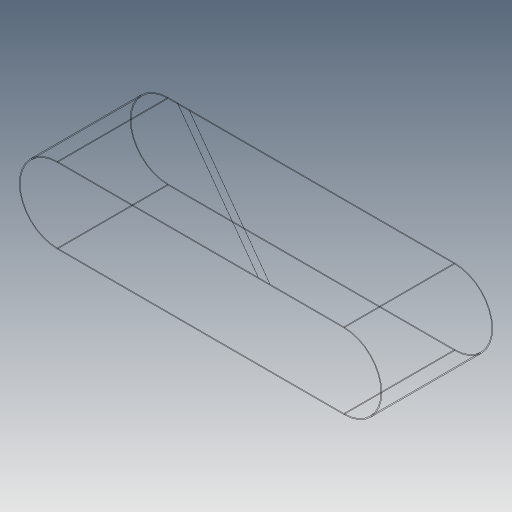
# Autodesk Inventor part: J005559
Saved by Autodesk Inventor 2023.3 (Build 273359000, 359)
## iProperties
RuleStatus: InUse
Created: 2015-04-28
Material: POLYESTER, BLACK
Vendor: HHMI: JRC - ID&F
Document SubType Name: Modeling
Designer: ARNOLDJ
Density: 1 g/cm^3
Appearance: Skid Plate
Description: RIBBON FLAT BELT
Project: COMMON
Part Number: J005559
AfterDocSave0: file://Part Number Cleaner
LAB/DEPT: COMMON
REQUESTING SCIENTIST: COMMON
SURFACE ROUGHNESS: N/A
DESIGN DEPARTMENT: HHMI: JRC - ID&F
SPECIAL FINISH: NONE
ALTERED ITEM PART NUMBER: SEE DRAWING
ALTERED ITEM VENDOR: SEE DRAWING
ALTERED ITEM DESCRIPTION: SEE DRAWING
Revision Number: B
Autodesk Inventor part; units mm, degrees
ref_plane "YZ Plane" through (0, 0, 0) normal (1, 0, 0) x (0, 1, 0)
ref_plane "XZ Plane" through (0, 0, 0) normal (0, 1, 0) x (-1, 0, 0)
ref_plane "XY Plane" through (0, 0, 0) normal (0, 0, 1) x (1, 0, 0)
sketch "Sketch1" plane through (0, 0, 0) normal (0, 0, 1) x (1, 0, 0)
  line L0 (0, 26.7405) -> (0, -19.6883) projected
  line L1 (-211.1375, 0) -> (211.1375, 0) projected
  arc A0 (-49.276, 12.9032) -> (-49.276, -12.9032) centre (-49.276, 0) ccw
  arc A1 (49.276, -12.9032) -> (49.276, 12.9032) centre (49.276, 0) ccw
  line L2 (0, 0) -> (0, 20.1078) construction
  line L3 (-49.276, 12.9032) -> (49.276, 12.9032)
  line L4 (-49.276, -12.9032) -> (49.276, -12.9032)
  line L5 (49.276, 13.0556) -> (-49.276, 13.0556)
  arc A2 (-49.276, 13.0556) -> (-49.276, -13.0556) centre (-49.276, 0) ccw
  line L6 (-49.276, -13.0556) -> (49.276, -13.0556)
  arc A3 (49.276, -13.0556) -> (49.276, 13.0556) centre (49.276, 0) ccw
  line L7 (49.276, 12.7508) -> (-49.276, 12.7508)
  arc A4 (-49.276, 12.7508) -> (-49.276, -12.7508) centre (-49.276, 0) ccw
  line L8 (-49.276, -12.7508) -> (49.276, -12.7508)
  arc A5 (49.276, -12.7508) -> (49.276, 12.7508) centre (49.276, 0) ccw
  dimension "d0" = 25.8064
  dimension "d1" = 98.552
  dimension "d2" = 12.9032
  dimension "d3" = 0.1524
  dimension "d4" = 0.1524
  dimension "d7" = 12.7508
  constraints: 14 end point, 12 point on circle, 6 centre point, 3 point on line, 2 tangent, 1 equal radius, 1 horizontal, 1 symmetric about line, 6 other
  measures "d0" diameter of A0
  measures "d1" distance of A1.centre A0.centre
  measures "d2" radius of A1
  measures "d3" distance between parallel lines of L5 L3
  measures "d4" distance between parallel lines of L3 L7
  measures "d7" radius of A4
extrude "Extrusion1" add sketch "Sketch1" along normal mid plane 38.1 contours L5 A3 L1 A1 L3 L0 | L0 L3 A0 L1 A2 L5 | L3 A1 L1 A5 L7 L0 | L0 L7 A4 L1 A0 L3 | A3 L6 L0 L4 A1 L1 | L1 A0 L4 L0 L6 A2 | L1 A4 L8 L0 L4 A0 | A1 L4 L0 L8 A5 L1
sketch "Sketch4" plane through (-49.276, 13.0556, 19.05) normal (0, 1, 0) x (1, 0, 0)
  line L0 (0, 38.1) -> (98.552, 38.1) projected
  line L1 (3.1607, 38.1) -> (69.1519, 0)
  line L2 (98.552, 0) -> (0, 0) projected
  line L3 (7.1607, 38.1) -> (73.1519, 0)
  point P0 (49.276, 19.05)
  dimension "d88" = 30
  dimension "d89" = 2
  constraints: 4 end point, 4 point on line, 1 parallel
  measures "d88" angle of L1 L0
  measures "d89" distance between parallel lines of L1 L3
extrude "Extrusion7" cut sketch "Sketch4" against normal blind 0.0254
body "Solid1"
